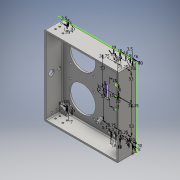
# Autodesk Inventor part: RcTransmitter
Saved by Autodesk Inventor 2016 (Build 200138000, 138)
## iProperties
Created: 2026-01-21
Part Number: RcTransmitter
Material: Generic
Document SubType Name: Modeling
Designer: Steve
Density: 1 g/cm^3
Appearance: Default
Author: Steve
Autodesk Inventor part; units mm, degrees
ref_plane "YZ Plane" through (0, 0, 0) normal (1, 0, 0) x (0, 1, 0)
ref_plane "XZ Plane" through (0, 0, 0) normal (0, 1, 0) x (-1, 0, 0)
ref_plane "XY Plane" through (0, 0, 0) normal (0, 0, 1) x (1, 0, 0)
sketch "Sketch1" plane through (0, 0, 0) normal (0, 1, 0) x (-1, 0, 0)
  line L0 (65, 75) -> (-75, 75)
  line L1 (-75, 75) -> (-75, -75)
  line L2 (-75, -75) -> (65, -75)
  line L3 (65, -75) -> (65, 75)
  circle A0 centre (25, 35) radius 25
  circle A1 centre (25, -35) radius 25
  circle A2 centre (47.5, 57.5) radius 1.6
  circle A3 centre (47.5, 12.5) radius 1.6
  circle A4 centre (2.5, 12.5) radius 1.6
  circle A5 centre (2.5, 57.5) radius 1.6
  circle A6 centre (47.5, -12.5) radius 1.6
  circle A7 centre (47.5, -57.5) radius 1.6
  circle A8 centre (2.5, -57.5) radius 1.6
  circle A9 centre (2.5, -12.5) radius 1.6
  point P0 (0, 0)
  dimension "d0" = 75
  dimension "d1" = 75
  dimension "d2" = 150
  dimension "d3" = 140
  dimension "d4" = 50
  dimension "d5" = 50
  dimension "d6" = 40
  dimension "d7" = 40
  dimension "d9" = 40
  dimension "d10" = 40
  dimension "d13" = 22.5
  dimension "d14" = 22.5
  dimension "d15" = 22.5
  dimension "d16" = 22.5
  dimension "d17" = 22.5
  dimension "d18" = 22.5
  dimension "d19" = 22.5
  dimension "d20" = 22.5
  dimension "d21" = 3.2
  dimension "d22" = 3.2
  dimension "d23" = 3.2
  dimension "d24" = 3.2
  dimension "d25" = 22.5
  dimension "d26" = 22.5
  dimension "d27" = 22.5
  dimension "d28" = 22.5
  dimension "d29" = 22.5
  dimension "d30" = 22.5
  dimension "d31" = 22.5
  dimension "d32" = 22.5
  dimension "d33" = 3.2
  dimension "d34" = 3.2
  dimension "d35" = 3.2
  dimension "d36" = 3.2
  constraints: 10 centre point, 8 end point, 2 parallel, 1 horizontal, 1 perpendicular
  measures "d0" distance from line of L2 point (0, 0)
  measures "d1" distance from line of L1 point (0, 0)
  measures "d2" distance of L2.end L0.start
  measures "d3" distance of L0.start L0.end
  measures "d4" diameter of A0
  measures "d5" diameter of A1
  measures "d6" distance from line of L2 A1.centre
  measures "d7" distance from line of L3 A1.centre
  measures "d9" distance from line of L0 A0.centre
  measures "d10" distance from line of L3 A0.centre
  measures "d13" horizontal distance of A2.centre A0.centre
  measures "d14" horizontal distance of A5.centre A0.centre
  measures "d15" horizontal distance of A3.centre A0.centre
  measures "d16" horizontal distance of A4.centre A0.centre
  measures "d17" horizontal distance of A5.centre A0.centre
  measures "d18" horizontal distance of A0.centre A4.centre
  measures "d19" horizontal distance of A0.centre A3.centre
  measures "d20" horizontal distance of A2.centre A0.centre
  measures "d21" diameter of A2
  measures "d22" diameter of A3
  measures "d23" diameter of A4
  measures "d24" diameter of A5
  measures "d25" horizontal distance of A6.centre A1.centre
  measures "d26" horizontal distance of A9.centre A1.centre
  measures "d27" horizontal distance of A9.centre A1.centre
  measures "d28" horizontal distance of A6.centre A1.centre
  measures "d29" horizontal distance of A7.centre A1.centre
  measures "d30" horizontal distance of A7.centre A1.centre
  measures "d31" horizontal distance of A8.centre A1.centre
  measures "d32" horizontal distance of A8.centre A1.centre
  measures "d33" diameter of A7
  measures "d34" diameter of A6
  measures "d35" diameter of A9
  measures "d36" diameter of A8
extrude "Extrusion2" add sketch "Sketch1" along normal blind 35
sketch "Sketch2" plane through (0, 0, 0) normal (0, -1, 0) x (1, 0, 0)
  line L0 (72, -72) -> (-62, -72)
  line L1 (-62, -72) -> (-62, 72)
  line L2 (-62, 72) -> (72, 72)
  line L3 (72, 72) -> (72, -72)
  line L4 (-65, 75) -> (75, 75) projected
  line L5 (75, 75) -> (75, -75) projected
  line L6 (75, -75) -> (-65, -75) projected
  line L7 (-65, -75) -> (-65, 75) projected
  point P0 (0, 0)
  dimension "d299" = 3
  dimension "d300" = 3
  dimension "d301" = 3
  dimension "d302" = 3
  constraints: 8 end point, 2 parallel, 1 horizontal, 1 perpendicular
  measures "d299" distance between parallel lines of L2 L4
  measures "d300" distance between parallel lines of L3 L5
  measures "d301" distance between parallel lines of L0 L6
  measures "d302" distance between parallel lines of L1 L7
extrude "Extrusion3" cut sketch "Sketch2" against normal blind 32 contours L0 L1 L2 L3
sketch "Sketch8" plane through (-65, 0, 75) normal (0, 0, 1) x (1, 0, 0)
  circle A0 centre (10, 19) radius 1.6
  circle A1 centre (10, 11) radius 1.6
  circle A2 centre (24, 19) radius 1.6
  circle A3 centre (24, 11) radius 1.6
  line L0 (0, 0) -> (0, 35) projected
  line L1 (0, 35) -> (140, 35) projected
  point P0 (110, 0)
  dimension "d169" = 3.2
  dimension "d170" = 3.2
  dimension "d171" = 3.2
  dimension "d172" = 3.2
  dimension "d179" = 14
  dimension "d180" = 14
  dimension "d355" = 10
  dimension "d356" = 8
  dimension "d357" = 8
  dimension "d368" = 16
  dimension "d369" = 16
  constraints: 4 centre point
  measures "d169" diameter of A2
  measures "d170" diameter of A3
  measures "d171" diameter of A1
  measures "d172" diameter of A0
  measures "d179" distance of A2.centre A0.centre
  measures "d180" distance of A3.centre A1.centre
  measures "d355" distance from line of L0 A1.centre
  measures "d356" distance of A2.centre A3.centre
  measures "d357" distance of A0.centre A1.centre
  measures "d368" distance from line of L1 A0.centre
  measures "d369" distance from line of L1 A2.centre
extrude "Extrusion7" cut sketch "Sketch8" against normal through all
sketch "Sketch9" plane through (-65, 0, -75) normal (-1, 0, 0) x (0, 0, 1)
  circle A0 centre (140, 19) radius 1.6
  circle A1 centre (140, 11) radius 1.6
  circle A2 centre (10, 19) radius 1.6
  circle A3 centre (10, 11) radius 1.6
  line L0 (150, 0) -> (150, 35) projected
  line L1 (0, 0) -> (0, 35) projected
  line L2 (0, 35) -> (150, 35) projected
  dimension "d183" = 3.2
  dimension "d186" = 3.2
  dimension "d188" = 3.2
  dimension "d189" = 3.2
  dimension "d358" = 8
  dimension "d359" = 8
  dimension "d360" = 10
  dimension "d361" = 10
  dimension "d362" = 10
  dimension "d363" = 10
  dimension "d366" = 16
  dimension "d367" = 16
  constraints: 4 centre point
  measures "d183" diameter of A2
  measures "d186" diameter of A3
  measures "d188" diameter of A0
  measures "d189" diameter of A1
  measures "d358" distance of A0.centre A1.centre
  measures "d359" distance of A2.centre A3.centre
  measures "d360" distance from line of L0 A1.centre
  measures "d361" distance from line of L0 A0.centre
  measures "d362" distance from line of L1 A3.centre
  measures "d363" distance from line of L1 A2.centre
  measures "d366" distance from line of L2 A2.centre
  measures "d367" distance from line of L2 A0.centre
sketch "Sketch11" plane through (0, 35, 0) normal (0, 1, 0) x (1, 0, 0)
  circle A0 centre (67, -67) radius 3
  circle A1 centre (67, -67) radius 1.75
  circle A2 centre (67, 67) radius 3.5
  circle A3 centre (67, 67) radius 1.75
  circle A4 centre (-57, -67) radius 3
  circle A5 centre (-57, -67) radius 1.75
  circle A6 centre (-57, 67) radius 3.5
  circle A7 centre (-57, 67) radius 1.75
  line L0 (-65, -75) -> (75, -75) projected
  line L1 (75, -75) -> (75, 75) projected
  line L2 (-65, 75) -> (-65, -75) projected
  line L3 (75, 75) -> (-65, 75) projected
  line L4 (72, -72) -> (72, 72) projected
  line L5 (72, -72) -> (62, -72)
  line L6 (62, -72) -> (62, -62)
  line L7 (62, -62) -> (72, -62)
  line L8 (72, -62) -> (72, -72)
  line L9 (72, 72) -> (62, 72)
  line L10 (62, 72) -> (62, 62)
  line L11 (62, 62) -> (72, 62)
  line L12 (72, 62) -> (72, 72)
  line L13 (-62, 72) -> (-62, -72) projected
  line L14 (-62, -72) -> (-52, -72)
  line L15 (-52, -72) -> (-52, -62)
  line L16 (-52, -62) -> (-62, -62)
  line L17 (-62, -62) -> (-62, -72)
  line L18 (-62, 72) -> (-52, 72)
  line L19 (-52, 72) -> (-52, 62)
  line L20 (-52, 62) -> (-62, 62)
  line L21 (-62, 62) -> (-62, 72)
  circle A8 centre (10, -53) radius 1.75
  circle A9 centre (64, -53) radius 1.75
  circle A10 centre (10, 53) radius 1.75
  circle A11 centre (64, 53) radius 1.75
  circle A12 centre (10, -53) radius 3
  circle A13 centre (64, -53) radius 3
  circle A14 centre (10, 53) radius 3
  circle A15 centre (64, 53) radius 3
  circle A16 centre (64, -53) radius 4.5
  circle A17 centre (10, -53) radius 4.5
  circle A18 centre (10, 53) radius 4.5
  circle A19 centre (64, 53) radius 4.5
  line L22 (23.75, -12) -> (16.75, -12)
  line L23 (16.75, -12) -> (16.75, 12)
  line L24 (16.75, 12) -> (23.75, 12)
  line L25 (23.75, 12) -> (23.75, -12)
  circle A20 centre (35, 65) radius 2.55
  circle A21 centre (45, 65) radius 2.55
  circle A22 centre (25, 65) radius 2.55
  circle A23 centre (45, -65) radius 2.55
  circle A24 centre (35, -65) radius 2.55
  circle A25 centre (25, -65) radius 2.55
  line L26 (75, 75) -> (-75, 75)
  line L27 (-75, -75) -> (75, -75)
  line L28 (75, -75) -> (75, 75)
  circle A26 centre (38.75, 20) radius 3.6
  circle A27 centre (38.75, 0) radius 3.6
  circle A28 centre (38.75, -20) radius 3.6
  point P0 (0, 0)
  point P1 (6.25, 0)
  dimension "d229" = 7
  dimension "d230" = 3.5
  dimension "d231" = 3.5
  dimension "d232" = 6
  dimension "d233" = 3.5
  dimension "d234" = 6
  dimension "d235" = 3.5
  dimension "d236" = 7
  dimension "d386" = 8
  dimension "d387" = 8
  dimension "d388" = 8
  dimension "d389" = 8
  dimension "d390" = 8
  dimension "d391" = 8
  dimension "d392" = 8
  dimension "d393" = 8
  dimension "d452" = 10
  dimension "d453" = 10
  dimension "d454" = 10
  dimension "d455" = 10
  dimension "d456" = 10
  dimension "d457" = 10
  dimension "d458" = 10
  dimension "d459" = 10
  dimension "d476" = 53
  dimension "d477" = 53
  dimension "d478" = 53
  dimension "d479" = 53
  dimension "d499" = 7
  dimension "d500" = 24
  dimension "d501" = 12
  dimension "d502" = 5.1
  dimension "d503" = 5.1
  dimension "d504" = 5.1
  dimension "d505" = 10
  dimension "d506" = 10
  dimension "d507" = 5.1
  dimension "d508" = 5.1
  dimension "d509" = 5.1
  dimension "d510" = 10
  dimension "d511" = 10
  dimension "d512" = 10
  dimension "d513" = 10
  dimension "d514" = 10
  dimension "d515" = 10
  dimension "d516" = 10
  dimension "d517" = 10
  dimension "d518" = 30
  dimension "d519" = 30
  dimension "d523" = 20
  dimension "d524" = 15
  dimension "d525" = 15
  dimension "d526" = 15
  dimension "d527" = 20
  dimension "d528" = 0
  dimension "d534" = 28.75
  dimension "d537" = 28.75
  dimension "d538" = 25.25
  dimension "d539" = 33.25
  dimension "d540" = 25.25
  constraints: 46 end point, 29 centre point, 12 coincident, 10 parallel, 5 horizontal, 5 perpendicular
  measures "d229" diameter of A2
  measures "d230" diameter of A3
  measures "d231" diameter of A1
  measures "d232" diameter of A0
  measures "d233" diameter of A5
  measures "d234" diameter of A4
  measures "d235" diameter of A7
  measures "d236" diameter of A6
  measures "d386" distance from line of L0 A0.centre
  measures "d387" distance from line of L1 A0.centre
  measures "d388" distance from line of L0 A4.centre
  measures "d389" distance from line of L2 A4.centre
  measures "d390" distance from line of L3 A6.centre
  measures "d391" distance from line of L2 A6.centre
  measures "d392" distance from line of L3 A2.centre
  measures "d393" distance from line of L1 A2.centre
  measures "d452" distance of L6.end L7.end
  measures "d453" distance of L5.end L6.end
  measures "d454" distance of L11.end L10.end
  measures "d455" distance of L10.end L9.end
  measures "d456" distance of L16.end L15.end
  measures "d457" distance of L15.end L14.end
  measures "d458" distance of L19.end L20.end
  measures "d459" distance of L18.end L19.end
  measures "d476" vertical distance of point (0, 0) A12.centre
  measures "d477" vertical distance of point (0, 0) A9.centre
  measures "d478" vertical distance of point (0, 0) A10.centre
  measures "d479" vertical distance of point (0, 0) A11.centre
  measures "d499" distance of L23.end L24.end
  measures "d500" distance of L22.end L23.end
  measures "d501" distance from line of point (6.25, 0) L24
  measures "d502" diameter of A22
  measures "d503" diameter of A20
  measures "d504" diameter of A21
  measures "d505" distance of A20.centre A21.centre
  measures "d506" distance of A20.centre A22.centre
  measures "d507" diameter of A23
  measures "d508" diameter of A24
  measures "d509" diameter of A25
  measures "d510" distance of A24.centre A23.centre
  measures "d511" distance of A25.centre A24.centre
  measures "d512" distance from line of L26 A22.centre
  measures "d513" distance from line of L26 A20.centre
  measures "d514" distance from line of L26 A21.centre
  measures "d515" distance from line of L27 A25.centre
  measures "d516" distance from line of L27 A24.centre
  measures "d517" distance from line of L27 A23.centre
  measures "d518" distance from line of L28 A23.centre
  measures "d519" distance from line of L28 A21.centre
  measures "d523" distance of A27.centre A26.centre
  measures "d524" distance from line of A26.centre L25
  measures "d525" distance from line of L25 A27.centre
  measures "d526" distance from line of L25 A28.centre
  measures "d527" distance of A28.centre A27.centre
  measures "d528" vertical distance of A27.centre point (6.25, 0)
  measures "d534" horizontal distance of A28.centre A8.centre
  measures "d537" horizontal distance of A14.centre A26.centre
  measures "d538" horizontal distance of A11.centre A26.centre
  measures "d539" distance from line of L4 A27.centre
  measures "d540" horizontal distance of A9.centre A28.centre
extrude "Extrusion21" cut sketch "Sketch9" against normal blind 10
sketch "Sketch16" plane through (-62, 0, 72) normal (1, 0, 0) x (0, 0, -1)
  circle A0 centre (72, 25) radius 3.25
  line L0 (144, 32) -> (0, 32) projected
  line L1 (144, 0) -> (0, 0) projected
  circle A1 centre (72, 10) radius 5.5
  point P0 (67, 0)
  point P1 (5, 32)
  point P2 (147, 0)
  point P3 (-3, 0)
  dimension "d370" = 6.5
  dimension "d412" = 75
  dimension "d413" = 75
  dimension "d431" = 11
  dimension "d432" = 15
  dimension "d433" = 7
  dimension "d434" = 10
  constraints: 2 centre point
  measures "d370" diameter of A0
  measures "d412" horizontal distance of point (147, 0) point (72, 25)
  measures "d413" horizontal distance of point (-3, 0) point (72, 25)
  measures "d431" diameter of A1
  measures "d432" distance of A1.centre point (72, 25)
  measures "d433" distance from line of L0 point (72, 25)
  measures "d434" distance from line of L1 A1.centre
extrude "Extrusion35" cut sketch "Sketch16" against normal blind 10
extrude "Extrusion40" add sketch "Sketch11" against normal blind 10 contours A0 | A1 | A2 | A3 | A4 | A5 | A6 | A7 | L5 L6 L7 L4 | L11 L10 L9 L4 | L18 L19 L20 L13 | L16 L15 L14 L13
extrude "Extrusion41" cut sketch "Sketch11" against normal blind 3 contours A0 | A2 | A4 | A6
extrude "Extrusion42" cut sketch "Sketch11" against normal through all contours A1 | A3 | A5 | A7
fillet "Fillet16" radius 5 12 edges at (-52, 28.5, -62) (62, 28.5, -62) (72, 28.5, -62) (62, 28.5, -72) (-52, 28.5, -72) (-62, 28.5, -62) (62, 28.5, 62) (72, 28.5, 62) (62, 28.5, 72) (-52, 28.5, 72) (-52, 28.5, 62) (-62, 28.5, 62)
fillet "Fillet17" radius 2 36 edges at (-50.5356, 32, -70.5356) (-52, 32, -67) (-53.4644, 32, -63.4644) (-57, 32, -62) (-60.5356, 32, -60.5356) (-62, 32, 0) (-60.5356, 32, 60.5356) (-57, 32, 62) (-53.4644, 32, 63.4644) (-52, 32, 67) (-50.5356, 32, 70.5356) (5, 32, 72) (62, 32, 67) (60.5356, 32, 70.5356) (67, 32, 62) (63.4644, 32, 63.4644) (70.5356, 32, 60.5356) (72, 32, 0) (67, 32, -62) (70.5356, 32, -60.5356) (62, 32, -67) (63.4644, 32, -63.4644) (60.5356, 32, -70.5356) (5, 32, -72) (-62, 12.5, -72) (-62, 12.5, 72) (72, 12.5, 72) (72, 12.5, -72) (75, 17.5, -75) (75, 35, 0) (5, 35, -75) (-65, 17.5, -75) (-65, 35, 0) (-65, 17.5, 75) (5, 35, 75) (75, 17.5, 75)
extrude "Extrusion43" add sketch "Sketch11" against normal blind 5 contours A16 | A17 | A18 | A19
extrude "Extrusion44" add sketch "Sketch11" against normal blind 10 contours A12 | A13 | A14 | A15
extrude "Extrusion45" cut sketch "Sketch11" against normal blind 3 contours A12 | A13 | A14 | A15
extrude "Extrusion46" cut sketch "Sketch11" against normal through all contours A8 | A9 | A10 | A11
fillet "Fillet18" radius 2 8 edges at (5.5, 32, -53) (7, 30, -53) (59.5, 32, -53) (61, 30, -53) (59.5, 32, 53) (61, 30, 53) (5.5, 32, 53) (7, 30, 53)
fillet "Fillet19" radius 2 4 edges at (5.5, 30, 53) (59.5, 30, 53) (59.5, 30, -53) (5.5, 30, -53)
extrude "Extrusion47" cut sketch "Sketch11" against normal through all contours L22 L23 L24 L25 | A20 | A21 | A22 | A23 | A24 | A25 | A26 | A27 | A28
body "Solid2"
